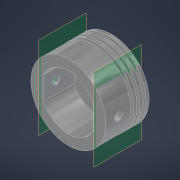
# Autodesk Inventor part: P003-Corps_piston
Saved by Autodesk Inventor 2021.3 (Build 253353000, 353)
## iProperties
Company: HES-SO
Created: 2022-03-18
Part Number: P003-Corps_piston
Material: Aluminium
Document SubType Name: Modeling
Designer: Rémi & Elise
Density: 2.7 g/cm^3
Appearance: Aluminum - Dark
Mass: 21.5358 g
Surface Area: 56.8938 cm^2
Volume: 7.9762 cm^3
Author: Rémi & Elise
Title: Corps piston
Autodesk Inventor part; units mm, degrees
ref_plane "XZ Plane" through (0, 0, 0) normal (0, 1, 0) x (-1, 0, 0)
ref_plane "XY Plane" through (0, 0, 0) normal (0, 0, 1) x (1, 0, 0)
sketch "Sketch5" plane through (0, 0, 0) normal (0, 0, 1) x (1, 0, 0)
  line L0 (-17.9489, 0) -> (2.9915, 0) construction
  line L1 (0, -3.44) -> (0, 20.64) construction
  line L2 (-10.9575, 0) -> (-10.9575, 12.2)
  line L3 (-10.9575, 12.2) -> (0, 12.2)
  line L4 (0, 17.2) -> (-14.9575, 17.2)
  line L5 (-14.9575, 17.2) -> (-14.9575, 16)
  line L6 (-14.9575, 16) -> (-12.9575, 16)
  line L7 (-12.9575, 16) -> (-12.9575, 14.8)
  line L8 (-12.9575, 14.8) -> (-14.9575, 14.8)
  line L9 (-14.9575, 14.8) -> (-14.9575, 13.6)
  line L10 (-14.9575, 13.6) -> (-12.9575, 13.6)
  line L11 (-12.9575, 13.6) -> (-12.9575, 12.4)
  line L12 (-12.9575, 12.4) -> (-14.9575, 12.4)
  line L13 (-14.9575, 12.4) -> (-14.9575, 11.2)
  line L14 (-14.9575, 11.2) -> (-12.9575, 11.2)
  line L15 (0, 17.2) -> (0, 12.2)
  line L16 (-12.9575, 11.2) -> (-12.9575, 10)
  line L17 (-12.9575, 10) -> (-14.9575, 10)
  line L18 (-14.9575, 10) -> (-14.9575, 0)
  line L19 (-14.9575, 0) -> (-10.9575, 0)
  point P0 (0, 0)
  dimension "d18" = 1.2
  dimension "d35" = 5
  dimension "d38" = 2
  dimension "d39" = 2
  dimension "d40" = 10
  dimension "d42" = 29.9149
  constraints: 36 end point, 11 perpendicular, 10 point on line, 5 parallel, 2 collinear, 2 vertical, 1 horizontal
  measures "d18" distance of L6.end L7.end
  measures "d35" distance of L4.start L3.end
  measures "d38" distance of L16.end L17.end
  measures "d39" distance between parallel lines of L2 L16
  measures "d40" distance of L17.end L18.end
  measures "d42" diameter of L5 L1
revolve "Revolution1" add sketch "Sketch5" angle 360 about axis through (0, -10, 0) along (0, 1, 0)
ref_plane "Work Plane1" through (20, 0, 0) normal (1, 0, 0) x (0, 1, 0)
sketch "Sketch6" plane through (20, 0, 0) normal (1, 0, 0) x (0, 1, 0)
  line L0 (11.2, -14.9575) -> (11.2, 14.9575) construction
  line L1 (12.4, -14.9575) -> (12.4, 14.9575) construction
  line L2 (13.6, -12.9575) -> (13.6, 12.9575) construction
  line L3 (13.6, -14.9575) -> (13.6, 14.9575) construction
  line L4 (14.8, -14.9575) -> (14.8, 14.9575) construction
  line L5 (14.8, -12.9575) -> (14.8, 12.9575) construction
  line L6 (16, -12.9575) -> (16, 12.9575) construction
  line L7 (16, -14.9575) -> (16, 14.9575) construction
  line L8 (17.2, -14.9575) -> (17.2, 14.9575) construction
  line L9 (-4.4, 0) -> (26.4, 0) construction
  line L10 (0, -14.9575) -> (0, 14.9575) construction
  point P0 (0, 0)
  point P1 (5, -17.5)
  point P2 (5, 17.5)
  point P3 (5, 0)
  dimension "d41" = 5
  constraints: 1 point on line
  measures "d41" distance from line of point (5, 0) L10
hole "Hole1" at (20, 5, 0) direction (-1, 0, 0) diameter 3 end through all
ref_plane "Work Plane3" through (10.9575, 6.1, 0) normal (-1, 0, 0) x (0, -1, 0)
ref_plane "Work Plane2" through (-14.2908, 5, 0) normal (-1, 0, 0) x (0, -0.4233179, 0.9059812)
sketch "Sketch7" plane through (10.9575, 6.1, 0) normal (-1, 0, 0) x (0, -1, 0)
  spline S0 degree 7 poles (-0.4, 0) (-0.4, -0.1802) (-0.3748, -0.3572) (-0.3258, -0.5267) (-0.2559, -0.6845) (-0.1685, -0.8273) (-0.0683, -0.953) (0.2813, -1.3027) (0.5706, -1.463) (0.8784, -1.5461) (1.1916, -1.5582) (1.5012, -1.5016) (1.7992, -1.369) (2.1855, -1.0487) (2.3082, -0.9188) (2.4168, -0.7663) (2.5049, -0.5936) (2.5674, -0.4047) (2.6, -0.2048) (2.6, 0.2049) (2.5674, 0.4048) (2.5049, 0.5936) (2.4168, 0.7663) (2.3082, 0.9188) (2.1856, 1.0487) (1.9351, 1.2559) (1.8054, 1.3383) (1.6696, 1.4034) (1.5298, 1.4518) (1.3874, 1.4839) (1.2437, 1.5) (0.9563, 1.5) (0.8126, 1.4839) (0.6702, 1.4518) (0.5304, 1.4034) (0.3946, 1.3383) (0.2649, 1.2559) (0.0145, 1.0487) (-0.1082, 0.9188) (-0.2168, 0.7663) (-0.305, 0.5936) (-0.3674, 0.4047) (-0.4, 0.2048) (-0.4, 0) knots 0 0 0 0 0 0 0 0 0.114256 0.114256 0.114256 0.114256 0.114256 0.114256 0.371167 0.371167 0.371167 0.371167 0.371167 0.371167 0.500252 0.500252 0.500252 0.500252 0.500252 0.500252 0.629363 0.629363 0.629363 0.629363 0.629363 0.629363 0.750149 0.750149 0.750149 0.750149 0.750149 0.750149 0.870934 0.870934 0.870934 0.870934 0.870934 0.870934 1 1 1 1 1 1 1 1 projected
  line L0 (6.1, 14.9575) -> (6.1, -14.9575) construction
  line L1 (-3.9, 14.9575) -> (-3.9, -14.9575) construction
  line L2 (-6.1, 6.1) -> (6.1, 6.1)
  line L3 (6.1, 6.1) -> (6.1, -6.1)
  line L4 (6.1, -6.1) -> (-6.1, -6.1)
  line L5 (-6.1, -6.1) -> (-6.1, 6.1)
  circle A0 centre (1.1, 0) radius 1.5 construction
  line L6 (-6.1, 10.9575) -> (-6.1, -10.9575) construction
  line L7 (-6.1, 6.1) -> (6.1, -6.1) construction
  line L8 (6.1, 6.1) -> (-6.1, -6.1) construction
  point P0 (6.1, 0)
  point P1 (0, 0)
  dimension "d43" = 3
  constraints: 12 end point, 3 perpendicular, 2 collinear, 2 parallel, 1 horizontal, 1 horizontal alignment, 1 midpoint, 2 other
  measures "d43" diameter of A0
extrude "Extrusion4" add sketch "Sketch7" along normal blind 1
ref_plane "Work Plane4" through (-10.9575, 0, 0) normal (-1, 0, 0) x (0, -1, 0)
sketch "Sketch8" plane through (-10.9575, 0, 0) normal (-1, 0, 0) x (0, -1, 0)
  line L0 (-12.2, 4.5733) -> (0, 4.5733) projected
  line L1 (-12.2, -4.5733) -> (-12.2, 4.5733) projected
  line L2 (0, -4.5733) -> (-12.2, -4.5733) projected
  line L3 (0, -4.5733) -> (0, 4.5733) projected
  circle A0 centre (-5, 0) radius 1.5 projected
  point P0 (0, 0)
extrude "Extrusion5" add sketch "Sketch8" against normal blind 1
body "Solid3"
